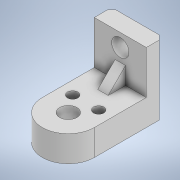
# Autodesk Inventor part: Деталь1
Saved by Autodesk Inventor 2022 (Build 260153000, 153)
## iProperties
Created: 2023-04-27
Part Number: Деталь1
Material: Типовые
Document SubType Name: Modeling
Designer: stasg
Density: 1 g/cm^3
Appearance: По умолчанию
Author: stasg
Autodesk Inventor part; units mm, degrees
ref_plane "YZ Plane" through (0, 0, 0) normal (1, 0, 0) x (0, 1, 0)
ref_plane "XZ Plane" through (0, 0, 0) normal (0, 1, 0) x (-1, 0, 0)
ref_plane "XY Plane" through (0, 0, 0) normal (0, 0, 1) x (1, 0, 0)
sketch "Эскиз1" plane through (0, 0, 0) normal (0, 1, 0) x (-1, 0, 0)
  line L0 (-5, 0) -> (-55, 0)
  line L1 (-60, 5) -> (-60, 80)
  line L2 (0, 80) -> (0, 5)
  arc A0 (0, 80) -> (-60, 80) centre (-30, 80) ccw
  circle A1 centre (-30, 80) radius 10
  circle A2 centre (-15, 60) radius 6
  circle A3 centre (-45, 60) radius 6
  line L3 (0, 5) -> (-5, 0)
  line L4 (-60, 5) -> (-55, 0)
  point P0 (0, 0)
  point P1 (-60, 0)
  dimension "d4" = 80
  dimension "d5" = 20
  dimension "d8" = 12
  dimension "d9" = 12
  dimension "d12" = 5
  dimension "d13" = 45
  dimension "d14" = 5
  dimension "d15" = 45
  constraints: 10 end point, 4 centre point, 4 point on line, 2 point on circle, 1 coincident, 1 horizontal, 1 parallel, 1 perpendicular
  measures "d4" distance of point (-60, 0) L1.end
  measures "d5" diameter of A1
  measures "d8" diameter of A2
  measures "d9" diameter of A3
  measures "d12" distance of L2.end point (0, 0)
  measures "d13" angle of L2 L3
  measures "d14" distance of L1.start point (-60, 0)
  measures "d15" angle of L1 L4
extrude "Выдавливание1" add sketch "Эскиз1" along normal blind 30
sketch "Эскиз2" plane through (0, 30, 0) normal (0, 1, 0) x (1, 0, 0)
  line L0 (0, -20) -> (60, -20)
  line L1 (60, -80) -> (60, -5) projected
  line L2 (60, -5) -> (55, 0) projected
  line L3 (60, -5) -> (55, 0)
  line L4 (55, 0) -> (5, 0) projected
  line L5 (55, 0) -> (5, 0)
  line L6 (5, 0) -> (0, -5) projected
  line L7 (5, 0) -> (0, -5)
  line L8 (0, -5) -> (0, -20)
  line L9 (0, -5) -> (0, -80) projected
  point P0 (0, 0)
  constraints: 10 end point, 4 collinear, 1 horizontal, 1 point on line
extrude "Выдавливание2" add sketch "Эскиз2" along normal blind 50
sketch "Эскиз3" plane through (0, 30, 20) normal (0, 0, 1) x (1, 0, 0)
  circle A0 centre (30, 35) radius 10
  line L0 (60, 0) -> (0, 0) projected
  point P0 (0, -30)
  dimension "d18" = 20
  constraints: 1 centre point
  measures "d18" diameter of A0
extrude "Выдавливание3" cut sketch "Эскиз3" against normal blind 50
ref_plane "РабПлоскость1" through (30, 0, 80) normal (1, 0, 0) x (0, 0, -1)
sketch "Эскиз6" plane through (30, 0, 80) normal (1, 0, 0) x (0, 0, -1)
  line L0 (60, 30) -> (0, 30) projected
  line L1 (40, 30) -> (60, 30)
  line L2 (60, 30) -> (60, 50)
  line L3 (60, 30) -> (60, 80) projected
  line L4 (60, 50) -> (40, 30)
  point P0 (80, 0)
  dimension "d26" = 20
  constraints: 6 end point, 2 point on line, 1 horizontal
  measures "d26" distance of L0.start L2.end
extrude "Выдавливание4" add sketch "Эскиз6" along normal mid plane 12
sketch "Эскиз7" plane through (0, 30, 0) normal (0, 1, 0) x (1, 0, 0)
  point P0 (0, 0)
equation "\"d14\" = d12"
equation "\"d15\" = d13"
